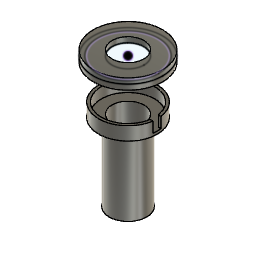
USonicHumidifier v1 (Autodesk Fusion 360 design; units mm, degrees)
Autodesk Fusion 360 part; units mm, degrees
note: some values were not read from the file. Set by a fixed rule: which sketch regions a step uses.
sketch "Sketch1" plane through (0, 0, 0) normal (0, 0, 1) x (1, 0, 0)
  circle A0 centre (0, 0) radius 10
  circle A1 centre (0, 0) radius 6
  circle A2 centre (0, 0) radius 11
  circle A3 centre (0, 0) radius 7
  line L0 (9.8869, -1.5) -> (10.8972, -1.5)
  line L1 (9.8869, 1.5) -> (10.8972, 1.5)
  dimension "d1" = 20
  dimension "d2" = 12
  constraint coincident A0.centre A1.centre
  constraint concentric A1 A2
  constraint concentric A0 A3
  constraint coincident A2 L1.end
  constraint coincident A0 L1.start
  constraint coincident A0 L0.start
  constraint coincident A2 L0.end
  measures "d1" diameter of A0
  measures "d2" diameter of A1
extrude "Extrude1" add sketch "Sketch1" against normal blind 30 contours A3 makes body 1
extrude "Extrude2" add sketch "Sketch1" against normal blind 1 contours A0 | A0 A2 L0 L1 | A0 A2 L0 L1 bodies 1
extrude "Extrude3" add sketch "Sketch1" along normal blind 4 contours A0 A2 L0 L1 | A0 A2 L0 L1 bodies 1
extrude "Extrude4" cut sketch "Sketch1" along normal blind 10.5 contours A0 A2 L0 L1 picked at (10.2446, 1.334) bodies 1
ref_plane "WorkPlane1" through (0, 0, 19) normal (0, 0, 1) x (1, 0, 0)
sketch "Sketch2" plane through (0, 0, 19) normal (0, 0, 1) x (1, 0, 0)
  circle A0 centre (0, 0) radius 11
  circle A1 centre (0, 0) radius 11.5
  circle A2 centre (0, 0) radius 13
  circle A3 centre (0, 0) radius 6
  dimension "d14" = 0.5
  dimension "d15" = 2
  dimension "d16" = 12
  constraint concentric A0 A3
  measures "d16" diameter of A3
extrude "Extrude5" add sketch "Sketch2" along normal blind 2 separate body contours A0 | A1 | A2 makes body 2
extrude "Extrude6" add sketch "Sketch2" against normal blind 2 contours A2 bodies 2
